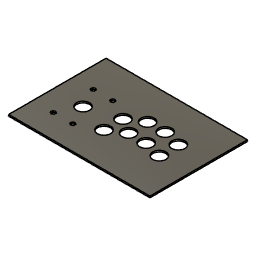
top2_hex (Autodesk Fusion 360 design; units mm, degrees)
Autodesk Fusion 360 part; units mm, degrees
sketch "Sketch2" plane through (0, 0, 73.1078) normal (0, 0, 1) x (-1, 0, 0)
  line L0 (112.9767, -87.8795) -> (112.9767, -92.4983)
  line L1 (112.9767, -92.4983) -> (108.9767, -94.8077)
  line L2 (108.9767, -94.8077) -> (104.9767, -92.4983)
  line L3 (104.9767, -92.4983) -> (104.9767, -87.8795)
  line L4 (104.9767, -87.8795) -> (108.9767, -85.5701)
  line L5 (108.9767, -85.5701) -> (112.9767, -87.8795)
  circle A0 centre (-4.5233, -88.1889) radius 13.5
  circle A1 centre (-76.5233, -40.1889) radius 13.5
  circle A2 centre (-4.5233, -49.1889) radius 13.5
  circle A3 centre (-40.5233, -88.1889) radius 13.5
  line L6 (72.9767, -92.4983) -> (68.9767, -94.8077)
  line L7 (68.9767, -94.8077) -> (64.9767, -92.4983)
  line L8 (64.9767, -92.4983) -> (64.9767, -87.8795)
  line L9 (64.9767, -87.8795) -> (68.9767, -85.5701)
  line L10 (68.9767, -85.5701) -> (72.9767, -87.8795)
  line L11 (72.9767, -87.8795) -> (72.9767, -92.4983)
  line L12 (64.9767, -10.4983) -> (64.9767, -5.8795)
  line L13 (64.9767, -5.8795) -> (68.9767, -3.5701)
  line L14 (68.9767, -3.5701) -> (72.9767, -5.8795)
  line L15 (72.9767, -5.8795) -> (72.9767, -10.4983)
  line L16 (72.9767, -10.4983) -> (68.9767, -12.8077)
  line L17 (68.9767, -12.8077) -> (64.9767, -10.4983)
  circle A4 centre (25.9767, -68.1889) radius 13.5
  circle A5 centre (-40.5233, -49.1889) radius 13.5
  circle A6 centre (25.9767, -29.1889) radius 13.5
  circle A7 centre (-76.5233, -79.1889) radius 13.5
  circle A8 centre (88.9767, -49.1889) radius 13.5
  line L18 (104.9767, -5.8795) -> (108.9767, -3.5701)
  line L19 (108.9767, -3.5701) -> (112.9767, -5.8795)
  line L20 (112.9767, -5.8795) -> (112.9767, -10.4983)
  line L21 (112.9767, -10.4983) -> (108.9767, -12.8077)
  line L22 (108.9767, -12.8077) -> (104.9767, -10.4983)
  line L23 (104.9767, -10.4983) -> (104.9767, -5.8795)
  line L24 (151.2267, 41.3111) -> (-138.7733, 41.3111)
  line L25 (-138.7733, 41.3111) -> (-138.7733, -158.6889)
  line L26 (-138.7733, -158.6889) -> (151.2267, -158.6889)
  line L27 (151.2267, -158.6889) -> (151.2267, 41.3111)
  circle A9 centre (88.9767, -49.1889) radius 13.5
  circle A10 centre (25.9767, -68.1889) radius 13.5
  circle A11 centre (-4.5233, -88.1889) radius 13.5
  circle A12 centre (-40.5233, -88.1889) radius 13.5
  circle A13 centre (-76.5233, -79.1889) radius 13.5
  circle A14 centre (-76.5233, -40.1889) radius 13.5
  circle A15 centre (-40.5233, -49.1889) radius 13.5
  circle A16 centre (-4.5233, -49.1889) radius 13.5
  circle A17 centre (25.9767, -29.1889) radius 13.5
  line L28 (108.9767, -3.5701) -> (104.9767, -5.8795)
  line L29 (104.9767, -5.8795) -> (104.9767, -10.4983)
  line L30 (104.9767, -10.4983) -> (108.9767, -12.8077)
  line L31 (108.9767, -12.8077) -> (112.9767, -10.4983)
  line L32 (112.9767, -10.4983) -> (112.9767, -5.8795)
  line L33 (112.9767, -5.8795) -> (108.9767, -3.5701)
  line L34 (108.9767, -12.8077) -> (112.9767, -10.4983)
  line L35 (112.9767, -10.4983) -> (112.9767, -5.8795)
  line L36 (112.9767, -5.8795) -> (108.9767, -3.5701)
  line L37 (108.9767, -3.5701) -> (104.9767, -5.8795)
  line L38 (104.9767, -5.8795) -> (104.9767, -10.4983)
  line L39 (104.9767, -10.4983) -> (108.9767, -12.8077)
  line L40 (108.9767, -3.5701) -> (108.9767, -3.5701)
  line L41 (108.9767, -3.5701) -> (108.9767, -3.5701)
  line L42 (108.9767, -3.5701) -> (108.9767, -3.5701)
  line L43 (108.9767, -3.5701) -> (108.9767, -3.5701)
  line L44 (108.9767, -3.5701) -> (108.9767, -3.5701)
  line L45 (108.9767, -3.5701) -> (108.9767, -3.5701)
  line L46 (68.9767, -3.5701) -> (64.9767, -5.8795)
  line L47 (64.9767, -5.8795) -> (64.9767, -10.4983)
  line L48 (64.9767, -10.4983) -> (68.9767, -12.8077)
  line L49 (68.9767, -12.8077) -> (72.9767, -10.4983)
  line L50 (72.9767, -10.4983) -> (72.9767, -5.8795)
  line L51 (72.9767, -5.8795) -> (68.9767, -3.5701)
  line L52 (68.9767, -12.8077) -> (72.9767, -10.4983)
  line L53 (72.9767, -10.4983) -> (72.9767, -5.8795)
  line L54 (72.9767, -5.8795) -> (68.9767, -3.5701)
  line L55 (68.9767, -3.5701) -> (64.9767, -5.8795)
  line L56 (64.9767, -5.8795) -> (64.9767, -10.4983)
  line L57 (64.9767, -10.4983) -> (68.9767, -12.8077)
  line L58 (68.9767, -3.5701) -> (68.9767, -3.5701)
  line L59 (68.9767, -3.5701) -> (68.9767, -3.5701)
  line L60 (68.9767, -3.5701) -> (68.9767, -3.5701)
  line L61 (68.9767, -3.5701) -> (68.9767, -3.5701)
  line L62 (68.9767, -3.5701) -> (68.9767, -3.5701)
  line L63 (68.9767, -3.5701) -> (68.9767, -3.5701)
  line L64 (68.9767, -85.5701) -> (64.9767, -87.8795)
  line L65 (64.9767, -87.8795) -> (64.9767, -92.4983)
  line L66 (64.9767, -92.4983) -> (68.9767, -94.8077)
  line L67 (68.9767, -94.8077) -> (72.9767, -92.4983)
  line L68 (72.9767, -92.4983) -> (72.9767, -87.8795)
  line L69 (72.9767, -87.8795) -> (68.9767, -85.5701)
  line L70 (68.9767, -94.8077) -> (72.9767, -92.4983)
  line L71 (72.9767, -92.4983) -> (72.9767, -87.8795)
  line L72 (72.9767, -87.8795) -> (68.9767, -85.5701)
  line L73 (68.9767, -85.5701) -> (64.9767, -87.8795)
  line L74 (64.9767, -87.8795) -> (64.9767, -92.4983)
  line L75 (64.9767, -92.4983) -> (68.9767, -94.8077)
  line L76 (68.9767, -85.5701) -> (68.9767, -85.5701)
  line L77 (68.9767, -85.5701) -> (68.9767, -85.5701)
  line L78 (68.9767, -85.5701) -> (68.9767, -85.5701)
  line L79 (68.9767, -85.5701) -> (68.9767, -85.5701)
  line L80 (68.9767, -85.5701) -> (68.9767, -85.5701)
  line L81 (68.9767, -85.5701) -> (68.9767, -85.5701)
  line L82 (108.9767, -85.5701) -> (104.9767, -87.8795)
  line L83 (104.9767, -87.8795) -> (104.9767, -92.4983)
  line L84 (104.9767, -92.4983) -> (108.9767, -94.8077)
  line L85 (108.9767, -94.8077) -> (112.9767, -92.4983)
  line L86 (112.9767, -92.4983) -> (112.9767, -87.8795)
  line L87 (112.9767, -87.8795) -> (108.9767, -85.5701)
  line L88 (108.9767, -94.8077) -> (112.9767, -92.4983)
  line L89 (112.9767, -92.4983) -> (112.9767, -87.8795)
  line L90 (112.9767, -87.8795) -> (108.9767, -85.5701)
  line L91 (108.9767, -85.5701) -> (104.9767, -87.8795)
  line L92 (104.9767, -87.8795) -> (104.9767, -92.4983)
  line L93 (104.9767, -92.4983) -> (108.9767, -94.8077)
  line L94 (108.9767, -85.5701) -> (108.9767, -85.5701)
  line L95 (108.9767, -85.5701) -> (108.9767, -85.5701)
  line L96 (108.9767, -85.5701) -> (108.9767, -85.5701)
  line L97 (108.9767, -85.5701) -> (108.9767, -85.5701)
  line L98 (108.9767, -85.5701) -> (108.9767, -85.5701)
  line L99 (108.9767, -85.5701) -> (108.9767, -85.5701)
  line L100 (151.2267, -158.6889) -> (-138.7733, -158.6889)
  line L101 (-138.7733, -158.6889) -> (-138.7733, 41.3111)
  line L102 (-138.7733, 41.3111) -> (151.2267, 41.3111)
  line L103 (151.2267, 41.3111) -> (151.2267, -158.6889)
  point P0 (108.9767, -8.1889)
  point P1 (108.9767, -8.1889)
  point P2 (108.9767, -3.5701)
  point P3 (68.9767, -8.1889)
  point P4 (68.9767, -8.1889)
  point P5 (68.9767, -3.5701)
  point P6 (68.9767, -90.1889)
  point P7 (68.9767, -90.1889)
  point P8 (68.9767, -85.5701)
  point P9 (108.9767, -90.1889)
  point P10 (108.9767, -90.1889)
  point P11 (108.9767, -85.5701)
  constraint concentric A8 A9
  constraint concentric A4 A10
  constraint concentric A0 A11
  constraint concentric A3 A12
  constraint concentric A7 A13
  constraint concentric A1 A14
  constraint concentric A5 A15
  constraint concentric A2 A16
  constraint concentric A6 A17
  constraint coincident P2 L18.end
  constraint coincident L18.start L23.end
  constraint coincident P5 L13.end
  constraint coincident L12.end L13.start
  constraint coincident P8 L9.end
  constraint coincident L8.end L9.start
  constraint coincident P11 L4.end
  constraint coincident L3.end L4.start
  constraint coincident L0.end L1.start
  constraint horizontal L100
  constraint vertical L101
  constraint horizontal L102
  constraint vertical L103
  constraint coincident L24.end L25.start
  constraint coincident L26.end L27.start
extrude "Extrude1" add sketch "Sketch2" along normal blind 3
equation "d150 = mat_thickness_3"
equation "mat_thickness_3 = 3 mm"
